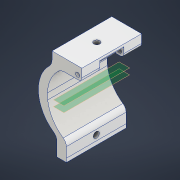
# Autodesk Inventor part: Part1
Saved by Autodesk Inventor 2021 (Build 250183000, 183)
## iProperties
Created: 2021-05-12
Part Number: Part1
Material: Aluminum 6061
Document SubType Name: Modeling
Designer: chick
Density: 2.7 g/cm^3
Appearance: Aluminum - Flat
Mass: 778.505 g
Surface Area: 509.833 cm^2
Volume: 288.335 cm^3
Author: chick
Autodesk Inventor part; units mm, degrees
ref_plane "YZ Plane" through (0, 0, 0) normal (1, 0, 0) x (0, 1, 0)
ref_plane "XZ Plane" through (0, 0, 0) normal (0, 1, 0) x (-1, 0, 0)
ref_plane "XY Plane" through (0, 0, 0) normal (0, 0, 1) x (1, 0, 0)
sketch "Sketch2" plane through (0, 0, 0) normal (0, 0, 1) x (1, 0, 0)
  line L0 (0, 20) -> (0, 0)
  line L1 (0, 0) -> (50, 0)
  line L2 (50, 0) -> (50, 20)
  line L3 (50, 20) -> (0, 20)
  dimension "base" = 20
  dimension "d1" = 50
  constraints: 8 end point, 3 perpendicular, 1 vertical
  measures "base" distance of L1.end L2.end
  measures "d1" distance of L2.end L0.start
extrude "Extrusion1" add sketch "Sketch2" along normal mid plane 100
sketch "Sketch12" plane through (0, 0, 50) normal (0, 0, 1) x (1, 0, 0)
  line L0 (24.0901, -129.6722) -> (24, -123.5405)
  line L1 (8.0901, -129.6722) -> (8.0901, -99.6722)
  line L2 (0, 0) -> (50, 0) projected
  arc A0 (0, 0) -> (8.0901, -99.6722) centre (37.1026, -47.1529) ccw
  line L3 (24, -123.5405) -> (24, -100)
  arc A1 (15, 0) -> (24, -100) centre (52.2273, -47.0545) ccw
  line L4 (8.0901, -129.6722) -> (24.0901, -129.6722)
  point P0 (24.2536, -50)
  dimension "d56" = 100
  dimension "d57" = 50
  dimension "d58" = 60
  dimension "d59" = 30
  dimension "d103" = 60
  dimension "d110" = 16
  dimension "d112" = 15
  constraints: 8 end point, 4 point on circle, 2 centre point, 2 vertical, 1 horizontal, 1 point on line
  measures "d56" distance of L1.end L2.start
  measures "d57" distance from line of point (24.254, -50) L2
  measures "d58" radius of A0
  measures "d59" distance of L1.start L1.end
  measures "d103" radius of A1
  measures "d110" distance of L1.start L0.start
  measures "d112" distance of L2.start A1.start
extrude "Extrusion6" add sketch "Sketch12" against normal blind 100
sketch "Sketch17" plane through (0, 0, 50) normal (0, 0, 1) x (1, 0, 0)
  line L0 (50, 0) -> (50, 20) projected
  line L1 (15, 0) -> (50, 0) projected
  circle A0 centre (43, 7) radius 3.5
  point P0 (0, 0)
  point P1 (10, 0)
  point P2 (43, 10.5)
  dimension "d84" = 7
  dimension "d82" = 7
  dimension "d83" = 7
  constraints: 1 coincident, 1 vertical alignment, 2 other
  measures "d82" distance from line of L0 point (43, 7)
  measures "d83" distance from line of L1 point (43, 7)
extrude "Extrusion8" cut sketch "Sketch17" against normal blind 100
sketch "Sketch18" plane through (50, 0, 50) normal (1, 0, 0) x (0, 0, -1)
  line L0 (0, 0) -> (100, 0) projected
  line L1 (30, 0) -> (70, 0)
  line L2 (0, 0) -> (0, 20) projected
  line L3 (30, 0) -> (30, 14)
  line L4 (30, 14) -> (70, 14)
  line L5 (0, 10.5) -> (100, 10.5) projected
  line L6 (70, 14) -> (70, 0)
  point P0 (50, 0)
  point P1 (70, 10.5)
  point P2 (30, 10.5)
  dimension "d104" = 14
  dimension "d105" = 20
  dimension "d106" = 20
  constraints: 8 end point, 2 point on line, 1 collinear, 1 parallel, 1 perpendicular, 1 vertical
  measures "d104" distance of L1.start L3.end
  measures "d105" distance from line of L6 point (50, 0)
  measures "d106" distance of L1.start point (50, 0)
extrude "Extrusion9" cut sketch "Sketch18" against normal blind 13 contours L3 L5 L6 L0 | L3 L4 L6 L5
sketch "Sketch19" plane through (8.0901, -129.6722, 50) normal (-1, 0, 0) x (0, 0, 1)
  line L0 (0, 0) -> (-100, 0) projected
  circle A0 centre (-50, 15) radius 5
  point P0 (-50, 129.6722)
  dimension "d91" = 15
  dimension "d92" = 10
  constraints: 1 centre point, 1 coincident
  measures "d91" distance from line of L0 point (-50, 15)
  measures "d92" diameter of A0
hole "Hole4" at (8.0901, -114.6722, 0) direction (1, 0, 0) diameter 10 end through all
fillet "Fillet1" radius 6 2 edges at (50, 0, 35) (50, 0, -35)
fillet "Fillet2" radius 16 1 edges at (0, 0, 0)
fillet "Fillet3" radius 16 1 edges at (15, 0, 0)
fillet "Fillet4" radius 12 2 edges at (8.0901, -99.6722, 0) (24, -100, 0)
fillet "Fillet5" radius 2 3 edges at (37, 14, 0) (50, 14, 0) (37, 0, 0)
ref_plane "Work Plane2" through (8.0901, -44.6722, 50) normal (0, -1, 0) x (1, 0, 0)
ref_plane "Work Plane3" through (8.0901, -54.6722, 50) normal (0, -1, 0) x (1, 0, 0)
split_face "Split3"
split_face "Split4"
sketch "Sketch20" plane through (0, 20, 50) normal (0, 1, 0) x (1, 0, 0)
  line L0 (0, 100) -> (0, 0) projected
  line L1 (50, 100) -> (50, 0) projected
  line L2 (0, 100) -> (50, 100) projected
  point P0 (0, 50)
  point P1 (25, 50)
  dimension "d116" = 50
  dimension "d117" = 100
  dimension "d118" = 50
  dimension "d119" = 25
  measures "d116" distance between parallel lines of L0 L1
  measures "d117" distance of L1.start L1.end
  measures "d118" distance from line of L2 point (25, 50)
  measures "d119" distance from line of L0 point (25, 50)
hole "Hole5" at (25, 20, 0) direction (0, -1, 0) diameter 10 depth 20 tip angle 118
equation "\"d56\" = arm_vertical_length"
equation "\"d59\" = connection_length"
equation "\"d103\" = d58"
equation "\"d105\" = d106"
equation "\"d118\" = 0.5 * d117"
equation "\"d119\" = 0.5 * d116"
equation "\"arm_thickness\" = 12"
equation "\"arm_vertical_length\" = 100"
equation "\"connection_length\" = 30"
body "Solid1"
